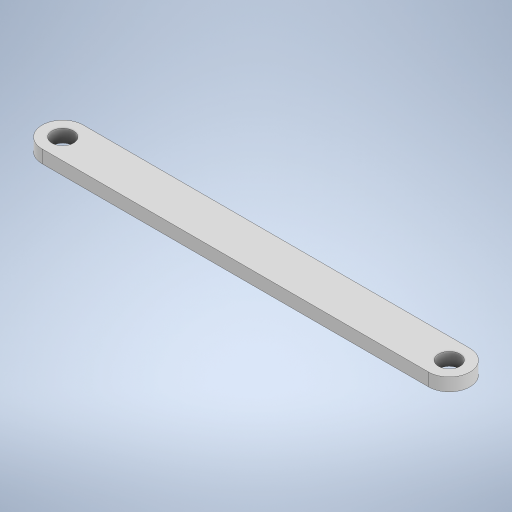
# Autodesk Inventor part: leg3
Saved by Autodesk Inventor 2024 (Build 280153000, 153)
## iProperties
Created: 2023-08-18
Part Number: leg3
Material: 常规
Document SubType Name: Modeling
Designer: wya
Density: 1 g/cm^3
Appearance: 默认
Author: wya
Autodesk Inventor part; units mm, degrees
ref_plane "YZ Plane" through (0, 0, 0) normal (1, 0, 0) x (0, 1, 0)
ref_plane "XZ Plane" through (0, 0, 0) normal (0, 1, 0) x (-1, 0, 0)
ref_plane "XY Plane" through (0, 0, 0) normal (0, 0, 1) x (1, 0, 0)
sketch "草图1" plane through (0, 0, 0) normal (0, 1, 0) x (-1, 0, 0)
  circle A0 centre (0, 0) radius 8
  line L0 (0, 8) -> (-150, 8)
  line L1 (-150, 8) -> (-150, -8)
  line L2 (-150, -8) -> (0, -8)
  line L3 (0, -8) -> (0, 8)
  circle A1 centre (0, 0) radius 4.15
  circle A2 centre (-150, 0) radius 8
  circle A3 centre (-150, 0) radius 4.15
  point P0 (-150, 8)
  dimension "d0" = 16
  dimension "d1" = 8.3
  dimension "d2" = 150
  dimension "d3" = 8.3
  constraints: 8 end point, 3 coincident, 2 centre point, 2 horizontal, 2 midpoint, 2 parallel, 1 perpendicular, 6 other
  measures "d0" distance between parallel lines of L2 L0
  measures "d1" diameter of A1
  measures "d2" distance between parallel lines of L1 L3
  measures "d3" diameter of A3
extrude "拉伸1" add sketch "草图1" along normal blind 5 contours A0 L3 A1 | L3 A1 A0 | A0 L2 A2 L0 | A2 L1 A3 | L1 A3 A2
